Autodesk Fusion 360 part; units mm, degrees
(part 2 of 2)
  spline S18 degree 5 poles (2.4575, 16.735) (2.4592, 16.7471) (2.4624, 16.7712) (2.466, 16.8075) (2.4685, 16.8561) (2.4687, 16.9171) (2.4667, 16.9782) (2.4633, 17.0395) (2.4593, 17.1009) (2.4548, 17.1623) (2.4497, 17.2237) (2.4439, 17.2852) (2.4372, 17.3467) (2.4294, 17.4083) (2.4206, 17.4699) (2.4107, 17.5316) (2.4, 17.5933) (2.3886, 17.6549) (2.3766, 17.7166) (2.364, 17.7783) (2.3508, 17.84) (2.337, 17.9017) (2.3225, 17.9634) (2.3073, 18.025) (2.2914, 18.0867) (2.2749, 18.1483) (2.2578, 18.2099) (2.2401, 18.2715) (2.2219, 18.3331) (2.2031, 18.3946) (2.1837, 18.4561) (2.1638, 18.5175) (2.1433, 18.579) (2.1223, 18.6403) (2.1007, 18.7017) (2.0786, 18.763) (2.056, 18.8242) (2.0329, 18.8854) (2.0092, 18.9465) (1.9851, 19.0076) (1.9605, 19.0686) (1.9353, 19.1296) (1.9097, 19.1905) (1.8836, 19.2514) (1.857, 19.3121) (1.8299, 19.3728) (1.8024, 19.4335) (1.7743, 19.494) (1.7459, 19.5545) (1.7169, 19.615) (1.6875, 19.6753) (1.6577, 19.7355) (1.6274, 19.7957) (1.5966, 19.8558) (1.5654, 19.9158) (1.5338, 19.9757) (1.5017, 20.0356) (1.4692, 20.0953) (1.4362, 20.155) (1.4029, 20.2145) (1.3691, 20.274) (1.3348, 20.3333) (1.3002, 20.3926) (1.2651, 20.4518) (1.2296, 20.5108) (1.1937, 20.5698) (1.1574, 20.6286) (1.1207, 20.6874) (1.0836, 20.746) (1.0461, 20.8045) (1.0082, 20.8629) (0.9775, 20.9095) (0.9544, 20.9445) (0.9388, 20.9677) (0.931, 20.9794) knots 0 0 0 0 0 0 0.01428571 0.02857143 0.04285714 0.05714286 0.07142857 0.08571429 0.1 0.11428571 0.12857143 0.14285714 0.15714286 0.17142857 0.18571429 0.2 0.21428571 0.22857143 0.24285714 0.25714286 0.27142857 0.28571429 0.3 0.31428571 0.32857143 0.34285714 0.35714286 0.37142857 0.38571429 0.4 0.41428571 0.42857143 0.44285714 0.45714286 0.47142857 0.48571429 0.5 0.51428571 0.52857143 0.54285714 0.55714286 0.57142857 0.58571429 0.6 0.61428571 0.62857143 0.64285714 0.65714286 0.67142857 0.68571429 0.7 0.71428571 0.72857143 0.74285714 0.75714286 0.77142857 0.78571429 0.8 0.81428571 0.82857143 0.84285714 0.85714286 0.87142857 0.88571429 0.9 0.91428571 0.92857143 0.94285714 0.95714286 0.97142857 0.98571429 1 1 1 1 1 1
  arc A29 (0.931, 20.9794) -> (-0.931, 20.9794) centre (0, 0) ccw
  spline S19 degree 5 poles (-0.931, 20.9794) (-0.9388, 20.9677) (-0.9544, 20.9445) (-0.9775, 20.9095) (-1.0082, 20.8629) (-1.0461, 20.8045) (-1.0836, 20.746) (-1.1207, 20.6874) (-1.1574, 20.6286) (-1.1937, 20.5698) (-1.2296, 20.5108) (-1.2651, 20.4518) (-1.3002, 20.3926) (-1.3348, 20.3333) (-1.3691, 20.274) (-1.4029, 20.2145) (-1.4362, 20.155) (-1.4692, 20.0953) (-1.5017, 20.0356) (-1.5338, 19.9757) (-1.5654, 19.9158) (-1.5966, 19.8558) (-1.6274, 19.7957) (-1.6577, 19.7355) (-1.6875, 19.6753) (-1.7169, 19.615) (-1.7459, 19.5545) (-1.7743, 19.494) (-1.8024, 19.4335) (-1.8299, 19.3728) (-1.857, 19.3121) (-1.8836, 19.2514) (-1.9097, 19.1905) (-1.9353, 19.1296) (-1.9605, 19.0686) (-1.9851, 19.0076) (-2.0092, 18.9465) (-2.0329, 18.8854) (-2.056, 18.8242) (-2.0786, 18.763) (-2.1007, 18.7017) (-2.1223, 18.6403) (-2.1433, 18.579) (-2.1638, 18.5175) (-2.1837, 18.4561) (-2.2031, 18.3946) (-2.2219, 18.3331) (-2.2401, 18.2715) (-2.2578, 18.2099) (-2.2749, 18.1483) (-2.2914, 18.0867) (-2.3073, 18.025) (-2.3225, 17.9634) (-2.337, 17.9017) (-2.3508, 17.84) (-2.364, 17.7783) (-2.3766, 17.7166) (-2.3886, 17.6549) (-2.4, 17.5933) (-2.4107, 17.5316) (-2.4206, 17.4699) (-2.4294, 17.4083) (-2.4372, 17.3467) (-2.4439, 17.2852) (-2.4497, 17.2237) (-2.4548, 17.1623) (-2.4593, 17.1009) (-2.4633, 17.0395) (-2.4667, 16.9782) (-2.4687, 16.9171) (-2.4685, 16.8561) (-2.466, 16.8075) (-2.4624, 16.7712) (-2.4592, 16.7471) (-2.4575, 16.735) knots -1 -1 -1 -1 -1 -1 -0.98571429 -0.97142857 -0.95714286 -0.94285714 -0.92857143 -0.91428571 -0.9 -0.88571429 -0.87142857 -0.85714286 -0.84285714 -0.82857143 -0.81428571 -0.8 -0.78571429 -0.77142857 -0.75714286 -0.74285714 -0.72857143 -0.71428571 -0.7 -0.68571429 -0.67142857 -0.65714286 -0.64285714 -0.62857143 -0.61428571 -0.6 -0.58571429 -0.57142857 -0.55714286 -0.54285714 -0.52857143 -0.51428571 -0.5 -0.48571429 -0.47142857 -0.45714286 -0.44285714 -0.42857143 -0.41428571 -0.4 -0.38571429 -0.37142857 -0.35714286 -0.34285714 -0.32857143 -0.31428571 -0.3 -0.28571429 -0.27142857 -0.25714286 -0.24285714 -0.22857143 -0.21428571 -0.2 -0.18571429 -0.17142857 -0.15714286 -0.14285714 -0.12857143 -0.11428571 -0.1 -0.08571429 -0.07142857 -0.05714286 -0.04285714 -0.02857143 -0.01428571 0 0 0 0 0 0
  line L19 (-2.4575, 16.735) -> (-2.2515, 15.3323)
  arc A30 (-3.0322, 14.2091) -> (-2.2515, 15.3323) centre (-3.2409, 15.1871) ccw
  arc A31 (-5.7163, 14.4039) -> (-4.4786, 13.8215) centre (-4.7868, 14.7728) ccw
  line L20 (-5.7163, 14.4039) -> (-6.2393, 15.7217)
  spline S20 degree 5 poles (-6.2393, 15.7217) (-6.2438, 15.733) (-6.2531, 15.7555) (-6.2682, 15.7887) (-6.2903, 15.8321) (-6.3206, 15.885) (-6.3529, 15.9369) (-6.3864, 15.9883) (-6.4206, 16.0394) (-6.4553, 16.0903) (-6.4904, 16.141) (-6.5261, 16.1914) (-6.5627, 16.2413) (-6.6002, 16.2907) (-6.6387, 16.3397) (-6.678, 16.3882) (-6.7181, 16.4362) (-6.7588, 16.4839) (-6.8001, 16.5314) (-6.8418, 16.5785) (-6.8841, 16.6253) (-6.927, 16.6718) (-6.9703, 16.718) (-7.0143, 16.7638) (-7.0589, 16.8092) (-7.104, 16.8544) (-7.1496, 16.8992) (-7.1957, 16.9436) (-7.2423, 16.9878) (-7.2894, 17.0317) (-7.3369, 17.0753) (-7.3849, 17.1185) (-7.4333, 17.1615) (-7.4822, 17.2042) (-7.5315, 17.2465) (-7.5813, 17.2885) (-7.6315, 17.3303) (-7.6822, 17.3717) (-7.7332, 17.4128) (-7.7847, 17.4536) (-7.8365, 17.4942) (-7.8888, 17.5344) (-7.9414, 17.5743) (-7.9944, 17.614) (-8.0479, 17.6533) (-8.1017, 17.6923) (-8.1559, 17.7311) (-8.2104, 17.7695) (-8.2653, 17.8077) (-8.3206, 17.8455) (-8.3762, 17.8831) (-8.4322, 17.9203) (-8.4885, 17.9573) (-8.5452, 17.9939) (-8.6022, 18.0303) (-8.6596, 18.0664) (-8.7173, 18.1022) (-8.7753, 18.1376) (-8.8337, 18.1728) (-8.8924, 18.2077) (-8.9514, 18.2423) (-9.0107, 18.2766) (-9.0703, 18.3106) (-9.1303, 18.3443) (-9.1905, 18.3777) (-9.2511, 18.4108) (-9.3119, 18.4436) (-9.3731, 18.4761) (-9.4345, 18.5084) (-9.4963, 18.5403) (-9.5583, 18.5719) (-9.6082, 18.597) (-9.6457, 18.6156) (-9.6708, 18.628) (-9.6834, 18.6342) knots 0 0 0 0 0 0 0.01428571 0.02857143 0.04285714 0.05714286 0.07142857 0.08571429 0.1 0.11428571 0.12857143 0.14285714 0.15714286 0.17142857 0.18571429 0.2 0.21428571 0.22857143 0.24285714 0.25714286 0.27142857 0.28571429 0.3 0.31428571 0.32857143 0.34285714 0.35714286 0.37142857 0.38571429 0.4 0.41428571 0.42857143 0.44285714 0.45714286 0.47142857 0.48571429 0.5 0.51428571 0.52857143 0.54285714 0.55714286 0.57142857 0.58571429 0.6 0.61428571 0.62857143 0.64285714 0.65714286 0.67142857 0.68571429 0.7 0.71428571 0.72857143 0.74285714 0.75714286 0.77142857 0.78571429 0.8 0.81428571 0.82857143 0.84285714 0.85714286 0.87142857 0.88571429 0.9 0.91428571 0.92857143 0.94285714 0.95714286 0.97142857 0.98571429 1 1 1 1 1 1
  arc A32 (-9.6834, 18.6342) -> (-11.296, 17.7031) centre (0, 0) ccw
  spline S21 degree 5 poles (-11.296, 17.7031) (-11.2969, 17.6892) (-11.2987, 17.6613) (-11.3013, 17.6194) (-11.3046, 17.5637) (-11.3082, 17.4942) (-11.3114, 17.4247) (-11.3143, 17.3554) (-11.3167, 17.2862) (-11.3187, 17.2171) (-11.3203, 17.1481) (-11.3215, 17.0792) (-11.3223, 17.0104) (-11.3227, 16.9418) (-11.3226, 16.8733) (-11.3222, 16.8049) (-11.3213, 16.7366) (-11.32, 16.6685) (-11.3183, 16.6005) (-11.3161, 16.5326) (-11.3136, 16.4649) (-11.3106, 16.3973) (-11.3072, 16.3299) (-11.3033, 16.2627) (-11.2991, 16.1955) (-11.2944, 16.1286) (-11.2892, 16.0618) (-11.2836, 15.9952) (-11.2776, 15.9287) (-11.2712, 15.8624) (-11.2643, 15.7963) (-11.2569, 15.7304) (-11.2491, 15.6646) (-11.2408, 15.5991) (-11.2321, 15.5337) (-11.223, 15.4685) (-11.2133, 15.4036) (-11.2032, 15.3388) (-11.1927, 15.2742) (-11.1816, 15.2099) (-11.1701, 15.1458) (-11.1581, 15.0819) (-11.1456, 15.0182) (-11.1327, 14.9548) (-11.1192, 14.8916) (-11.1052, 14.8286) (-11.0907, 14.766) (-11.0758, 14.7035) (-11.0603, 14.6413) (-11.0443, 14.5794) (-11.0278, 14.5178) (-11.0107, 14.4565) (-10.993, 14.3955) (-10.9747, 14.3348) (-10.9559, 14.2745) (-10.9365, 14.2145) (-10.9165, 14.1547) (-10.8961, 14.0953) (-10.8751, 14.0362) (-10.8535, 13.9774) (-10.8312, 13.9191) (-10.8081, 13.8613) (-10.7841, 13.8041) (-10.7591, 13.7475) (-10.7334, 13.6913) (-10.707, 13.6356) (-10.6803, 13.5801) (-10.6531, 13.525) (-10.6253, 13.4703) (-10.5965, 13.4163) (-10.5658, 13.3636) (-10.5393, 13.3228) (-10.5181, 13.2931) (-10.5033, 13.2738) (-10.4957, 13.2642) knots -1 -1 -1 -1 -1 -1 -0.98571429 -0.97142857 -0.95714286 -0.94285714 -0.92857143 -0.91428571 -0.9 -0.88571429 -0.87142857 -0.85714286 -0.84285714 -0.82857143 -0.81428571 -0.8 -0.78571429 -0.77142857 -0.75714286 -0.74285714 -0.72857143 -0.71428571 -0.7 -0.68571429 -0.67142857 -0.65714286 -0.64285714 -0.62857143 -0.61428571 -0.6 -0.58571429 -0.57142857 -0.55714286 -0.54285714 -0.52857143 -0.51428571 -0.5 -0.48571429 -0.47142857 -0.45714286 -0.44285714 -0.42857143 -0.41428571 -0.4 -0.38571429 -0.37142857 -0.35714286 -0.34285714 -0.32857143 -0.31428571 -0.3 -0.28571429 -0.27142857 -0.25714286 -0.24285714 -0.22857143 -0.21428571 -0.2 -0.18571429 -0.17142857 -0.15714286 -0.14285714 -0.12857143 -0.11428571 -0.1 -0.08571429 -0.07142857 -0.05714286 -0.04285714 -0.02857143 -0.01428571 0 0 0 0 0 0
  line L21 (-10.4957, 13.2642) -> (-9.616, 12.1524)
  arc A33 (-9.7305, 10.7893) -> (-9.616, 12.1524) centre (-10.4002, 11.5319) ccw
  arc A34 (-12.1524, 9.616) -> (-10.7893, 9.7305) centre (-11.5319, 10.4002) ccw
  line L22 (-12.1524, 9.616) -> (-13.2642, 10.4957)
  spline S22 degree 5 poles (-13.2642, 10.4957) (-13.2738, 10.5033) (-13.2931, 10.5181) (-13.3228, 10.5393) (-13.3636, 10.5658) (-13.4163, 10.5965) (-13.4703, 10.6253) (-13.525, 10.6531) (-13.5801, 10.6803) (-13.6356, 10.707) (-13.6913, 10.7334) (-13.7475, 10.7591) (-13.8041, 10.7841) (-13.8613, 10.8081) (-13.9191, 10.8312) (-13.9774, 10.8535) (-14.0362, 10.8751) (-14.0953, 10.8961) (-14.1547, 10.9165) (-14.2145, 10.9365) (-14.2745, 10.9559) (-14.3348, 10.9747) (-14.3955, 10.993) (-14.4565, 11.0107) (-14.5178, 11.0278) (-14.5794, 11.0443) (-14.6413, 11.0603) (-14.7035, 11.0758) (-14.766, 11.0907) (-14.8286, 11.1052) (-14.8916, 11.1192) (-14.9548, 11.1327) (-15.0182, 11.1456) (-15.0819, 11.1581) (-15.1458, 11.1701) (-15.2099, 11.1816) (-15.2742, 11.1927) (-15.3388, 11.2032) (-15.4036, 11.2133) (-15.4685, 11.223) (-15.5337, 11.2321) (-15.5991, 11.2408) (-15.6646, 11.2491) (-15.7304, 11.2569) (-15.7963, 11.2643) (-15.8624, 11.2712) (-15.9287, 11.2776) (-15.9952, 11.2836) (-16.0618, 11.2892) (-16.1286, 11.2944) (-16.1955, 11.2991) (-16.2627, 11.3033) (-16.3299, 11.3072) (-16.3973, 11.3106) (-16.4649, 11.3136) (-16.5326, 11.3161) (-16.6005, 11.3183) (-16.6685, 11.32) (-16.7366, 11.3213) (-16.8049, 11.3222) (-16.8733, 11.3226) (-16.9418, 11.3227) (-17.0104, 11.3223) (-17.0792, 11.3215) (-17.1481, 11.3203) (-17.2171, 11.3187) (-17.2862, 11.3167) (-17.3554, 11.3143) (-17.4247, 11.3114) (-17.4942, 11.3082) (-17.5637, 11.3046) (-17.6194, 11.3013) (-17.6613, 11.2987) (-17.6892, 11.2969) (-17.7031, 11.296) knots 0 0 0 0 0 0 0.01428571 0.02857143 0.04285714 0.05714286 0.07142857 0.08571429 0.1 0.11428571 0.12857143 0.14285714 0.15714286 0.17142857 0.18571429 0.2 0.21428571 0.22857143 0.24285714 0.25714286 0.27142857 0.28571429 0.3 0.31428571 0.32857143 0.34285714 0.35714286 0.37142857 0.38571429 0.4 0.41428571 0.42857143 0.44285714 0.45714286 0.47142857 0.48571429 0.5 0.51428571 0.52857143 0.54285714 0.55714286 0.57142857 0.58571429 0.6 0.61428571 0.62857143 0.64285714 0.65714286 0.67142857 0.68571429 0.7 0.71428571 0.72857143 0.74285714 0.75714286 0.77142857 0.78571429 0.8 0.81428571 0.82857143 0.84285714 0.85714286 0.87142857 0.88571429 0.9 0.91428571 0.92857143 0.94285714 0.95714286 0.97142857 0.98571429 1 1 1 1 1 1
  arc A35 (-17.7031, 11.296) -> (-18.6342, 9.6834) centre (0, 0) ccw
  spline S23 degree 5 poles (-18.6342, 9.6834) (-18.628, 9.6708) (-18.6156, 9.6457) (-18.597, 9.6082) (-18.5719, 9.5583) (-18.5403, 9.4963) (-18.5084, 9.4345) (-18.4761, 9.3731) (-18.4436, 9.3119) (-18.4108, 9.2511) (-18.3777, 9.1905) (-18.3443, 9.1303) (-18.3106, 9.0703) (-18.2766, 9.0107) (-18.2423, 8.9514) (-18.2077, 8.8924) (-18.1728, 8.8337) (-18.1376, 8.7753) (-18.1022, 8.7173) (-18.0664, 8.6596) (-18.0303, 8.6022) (-17.9939, 8.5452) (-17.9573, 8.4885) (-17.9203, 8.4322) (-17.8831, 8.3762) (-17.8455, 8.3206) (-17.8077, 8.2653) (-17.7695, 8.2104) (-17.7311, 8.1559) (-17.6923, 8.1017) (-17.6533, 8.0479) (-17.614, 7.9944) (-17.5743, 7.9414) (-17.5344, 7.8888) (-17.4942, 7.8365) (-17.4536, 7.7847) (-17.4128, 7.7332) (-17.3717, 7.6822) (-17.3303, 7.6315) (-17.2885, 7.5813) (-17.2465, 7.5315) (-17.2042, 7.4822) (-17.1615, 7.4333) (-17.1185, 7.3849) (-17.0753, 7.3369) (-17.0317, 7.2894) (-16.9878, 7.2423) (-16.9436, 7.1957) (-16.8992, 7.1496) (-16.8544, 7.104) (-16.8092, 7.0589) (-16.7638, 7.0143) (-16.718, 6.9703) (-16.6718, 6.927) (-16.6253, 6.8841) (-16.5785, 6.8418) (-16.5314, 6.8001) (-16.4839, 6.7588) (-16.4362, 6.7181) (-16.3882, 6.678) (-16.3397, 6.6387) (-16.2907, 6.6002) (-16.2413, 6.5627) (-16.1914, 6.5261) (-16.141, 6.4904) (-16.0903, 6.4553) (-16.0394, 6.4206) (-15.9883, 6.3864) (-15.9369, 6.3529) (-15.885, 6.3206) (-15.8321, 6.2903) (-15.7887, 6.2682) (-15.7555, 6.2531) (-15.733, 6.2438) (-15.7217, 6.2393) knots -1 -1 -1 -1 -1 -1 -0.98571429 -0.97142857 -0.95714286 -0.94285714 -0.92857143 -0.91428571 -0.9 -0.88571429 -0.87142857 -0.85714286 -0.84285714 -0.82857143 -0.81428571 -0.8 -0.78571429 -0.77142857 -0.75714286 -0.74285714 -0.72857143 -0.71428571 -0.7 -0.68571429 -0.67142857 -0.65714286 -0.64285714 -0.62857143 -0.61428571 -0.6 -0.58571429 -0.57142857 -0.55714286 -0.54285714 -0.52857143 -0.51428571 -0.5 -0.48571429 -0.47142857 -0.45714286 -0.44285714 -0.42857143 -0.41428571 -0.4 -0.38571429 -0.37142857 -0.35714286 -0.34285714 -0.32857143 -0.31428571 -0.3 -0.28571429 -0.27142857 -0.25714286 -0.24285714 -0.22857143 -0.21428571 -0.2 -0.18571429 -0.17142857 -0.15714286 -0.14285714 -0.12857143 -0.11428571 -0.1 -0.08571429 -0.07142857 -0.05714286 -0.04285714 -0.02857143 -0.01428571 0 0 0 0 0 0
  line L23 (-15.7217, 6.2393) -> (-14.4039, 5.7163)
  arc A36 (-13.8215, 4.4786) -> (-14.4039, 5.7163) centre (-14.7728, 4.7868) ccw
  circle A37 centre (0, 0) radius 10 construction
  circle A38 centre (-10, 0) radius 2
  arc A39 (-14.2091, -3.0322) -> (-13.8215, -4.4786) centre (0, 0) ccw
  arc A40 (-10.7893, -9.7305) -> (-9.7305, -10.7893) centre (0, 0) ccw
  arc A41 (-4.4786, -13.8215) -> (-3.0322, -14.2091) centre (0, 0) ccw
  arc A42 (3.0322, -14.2091) -> (4.4786, -13.8215) centre (0, 0) ccw
  arc A43 (9.7305, -10.7893) -> (10.7893, -9.7305) centre (0, 0) ccw
  arc A44 (13.8215, -4.4786) -> (14.2091, -3.0322) centre (0, 0) ccw
  arc A45 (14.2091, 3.0322) -> (13.8215, 4.4786) centre (0, 0) ccw
  arc A46 (10.7893, 9.7305) -> (9.7305, 10.7893) centre (0, 0) ccw
  arc A47 (4.4786, 13.8215) -> (3.0322, 14.2091) centre (0, 0) ccw
  arc A48 (-3.0322, 14.2091) -> (-4.4786, 13.8215) centre (0, 0) ccw
  arc A49 (-9.7305, 10.7893) -> (-10.7893, 9.7305) centre (0, 0) ccw
  circle A50 centre (0, 0) radius 1.75
  circle A51 centre (0, 0) radius 3.5
  line L24 (-10, -4) -> (36, -4)
  arc A52 (36, -4) -> (36, 4) centre (36, 0) ccw
  line L25 (36, 4) -> (-10, 4)
  arc A53 (-10, 4) -> (-10, -4) centre (-10, 0) ccw
  line L26 (-10, 0) -> (36, 0) construction
  circle A54 centre (36, 0) radius 2
  dimension "d15" = 20
  dimension "d16" = 4
  dimension "d25" = 7
  dimension "d27" = 8
  dimension "d28" = 4
  dimension "d206" = 46
  constraint coincident A0.centre A2.centre
  constraint coincident A37 A38.centre
  constraint tangent L24 A52
  constraint tangent A52 L25
  constraint parallel L24 L25
  constraint tangent L25 A53
  constraint tangent L24 A53
  constraint horizontal L26
  constraint coincident A38.centre A53.centre
  constraint concentric A52 A54
  measures "d15" diameter of A37
  measures "d16" diameter of A38
  measures "d25" diameter of A51
  measures "d27" diameter of A52
  measures "d28" diameter of A54
  measures "d206" distance of A38.centre A52.centre
extrude "Extrude4" add sketch "Connecting Rod" along normal blind 5 separate body contours A19 L12 S12 A20 S13 L13 A21 A44 A45 L24 A52 L25 | A19 L12 S12 A20 S13 L13 A21 A44 A45 L24 L25 A53 | A50 | A51 makes body 2
extrude "Extrude5" cut sketch "Connecting Rod" against normal blind 3 contours A51 bodies 1
sketch "Slider" plane through (0, 0, 8) normal (0, 0, 1) x (-1, 0, 0)
  line L0 (32, 5) -> (47, 5)
  line L1 (47, 5) -> (47, -5)
  line L2 (47, -5) -> (32, -5)
  line L3 (32, -5) -> (32, 5)
  circle A0 centre (36, 0) radius 2
  point P0 (36, 0)
  dimension "d33" = 10
  dimension "d34" = 15
  dimension "d209" = 4
  constraint horizontal L0
  constraint vertical L1
  constraint horizontal L2
  constraint vertical L3
  measures "d33" distance of L0.end L1.end
  measures "d34" distance of L0.start L0.end
  measures "d209" distance of L3 P0
extrude "Extrude6" add sketch "Slider" against normal blind 8 separate body makes body 3
extrude "Extrude7" add sketch "Connecting Rod" against normal blind 8 contours A54 bodies 3
extrude "Extrude8" add sketch "Connecting Rod" along normal blind 5 contours A38 bodies 1
extrude "Extrude9" add sketch "Connecting Rod" along normal blind 5 contours A54 bodies 3
sketch "Slider Dowel Hole" plane through (-47, 0, 0) normal (-1, 0, 0) x (0, -1, 0)
  line L0 (5, 8) -> (-5, 8)
  line L1 (-5, 8) -> (-5, 0)
  line L2 (-5, 0) -> (5, 0)
  line L3 (5, 0) -> (5, 8)
  line L4 (0, 1.75) -> (0, 22.5)
  circle A0 centre (0, 4) radius 3.1
  point P0 (2.2515, 8)
  dimension "d44" = 6.2
  dimension "d45" = 4
  constraint coincident L4 A0.centre
  measures "d44" diameter of A0
  measures "d45" vertical distance of A0.centre P0
extrude "Extrude10" cut sketch "Slider Dowel Hole" against normal blind 10 contours A0 bodies 3
sketch "Sketch17" plane through (-37, 0, 0) normal (-1, 0, 0) x (0, -1, 0)
  circle A0 centre (0, 4) radius 3.1
  circle A1 centre (0, 4) radius 3.1
  circle A2 centre (0, 4) radius 2.25
  dimension "d213" = 4.5
  constraint concentric A1 A2
  measures "d213" diameter of A2
extrude "Extrude26" cut sketch "Sketch17" against normal blind 5 contours A2 bodies 3
sketch "Connector Rod Clearance" plane through (0, 0, 13) normal (0, 0, 1) x (-1, 0, 0)
  circle A0 centre (-10, 0) radius 2
  circle A1 centre (36, 0) radius 2
  arc A2 (-10, 4) -> (-10, -4) centre (-10, 0) ccw
  line L0 (-10, -4) -> (36, -4)
  arc A3 (36, -4) -> (36, 4) centre (36, 0) ccw
  line L1 (36, 4) -> (-10, 4)
  circle A4 centre (-10, 0) radius 2
  circle A5 centre (36, 0) radius 2
  circle A6 centre (-10, 0) radius 2.15
  circle A7 centre (36, 0) radius 2.15
  dimension "d174" = 4.3
  dimension "d175" = 4.3
  constraint concentric A0 A6
  constraint concentric A1 A7
  measures "d174" diameter of A6
  measures "d175" diameter of A7
ref_plane "WorkPlane1" through (-36, 0, 13.5) normal (0, 0, 1) x (-1, 0, 0)
sketch "Sketch16" plane through (0, 0, 13.5) normal (0, 0, 1) x (1, 0, 0)
  circle A0 centre (-36, 0) radius 2
  circle A1 centre (-36, 0) radius 3
  circle A2 centre (10, 0) radius 2
  circle A3 centre (10, 0) radius 3
  dimension "d187" = 6
  dimension "d188" = 6
  constraint concentric A0 A1
  constraint concentric A2 A3
  measures "d187" diameter of A1
  measures "d188" diameter of A3
extrude "Extrude22" cut sketch "Connector Rod Clearance" against normal blind 5 contours A6 | A7 bodies 2
extrude "Extrude23" add sketch "Sketch16" along normal blind 4 separate body contours A0 | A1 | A2 | A3 makes body 4 at (-33.0149, -0.2987, 14.8333) makes body 5 at (12.9851, -0.2987, 14.8333)
extrude "Extrude24" cut sketch "Connector Rod Clearance" 2 faces at (9.427, 0.4727, 13) (-36.0487, -0.65, 13) along normal blind 2 contours A6 | A7 on bodies 1 3 bodies 4 5
extrude "Extrude33" add 1 faces at (-36.0487, -0.65, 13) along direction (0, 0, 1) blind 2 on bodies 3 bodies 3
extrude "Extrude34" add 1 faces at (9.427, 0.4727, 13) along direction (0, 0, 1) blind 2 on bodies 1 bodies 1
sketch "Base Plate" plane through (0, 0, 0) normal (0, 0, 1) x (1, 0, 0)
  line L0 (30, -25) -> (-71, -25)
  line L1 (-71, -25) -> (-71, 39)
  line L2 (30, 39) -> (30, -25)
  line L3 (-47, -5) -> (-47, 5)
  line L4 (0, 0) -> (17, 0) construction
  circle A0 centre (0, 0) radius 1.5
  line L5 (-22, -5.3) -> (-70, -5.3)
  line L6 (-70, -5.3) -> (-70, -10.3)
  line L7 (-70, -10.3) -> (-22, -10.3)
  line L8 (-22, -10.3) -> (-22, -5.3)
  line L9 (-32, -5) -> (-47, -5)
  line L10 (-32, 5) -> (-32, -5)
  line L11 (-22, 5.3) -> (-70, 5.3)
  line L12 (-70, 5.3) -> (-70, 10.3)
  line L13 (-70, 10.3) -> (-22, 10.3)
  line L14 (-22, 10.3) -> (-22, 5.3)
  line L15 (-71, 7) -> (-102, 7) construction
  line L16 (-20.5, 39) -> (-20.5, -25) construction
  line L17 (10, 0) -> (-36, 0) construction
  line L18 (0, 0) -> (9.2345, 25.3717) construction
  line L19 (0, 0) -> (27, 0) construction
  circle A1 centre (9.2345, 25.3717) radius 1.5
  line L20 (-71, 39) -> (30, 39)
  line L21 (-23.5, -3.8) -> (-30.5, -3.8)
  line L22 (-30.5, -3.8) -> (-30.5, 3.8)
  line L23 (-30.5, 3.8) -> (-23.5, 3.8)
  line L24 (-23.5, 3.8) -> (-23.5, -3.8)
  line L25 (-71, 39) -> (-71, 7) construction
  line L26 (-71, 29) -> (-72.5, 29)
  line L27 (-72.5, 29) -> (-72.5, 17)
  line L28 (-72.5, 17) -> (-71, 17)
  line L29 (-71, 17) -> (-71, 29)
  line L30 (30, -15) -> (31.5, -15)
  line L31 (31.5, -15) -> (31.5, -3)
  line L32 (31.5, -3) -> (30, -3)
  line L33 (30, -3) -> (30, -15)
  circle A2 centre (9.2345, 25.3717) radius 12 construction
  arc A3 (20.9794, -0.931) -> (20.9794, 0.931) centre (0, 0) ccw
  dimension "d48" = 25
  dimension "d53" = 3
  dimension "d55" = 0.3
  dimension "d57" = 10
  dimension "d59" = 5
  dimension "d198" = 27
  dimension "d199" = 70
  dimension "d200" = 3
  dimension "d210" = 23
  dimension "d211" = 1
  dimension "d216" = 1.5
  dimension "d217" = 1.5
  dimension "d218" = 1.5
  dimension "d219" = 1.5
  dimension "d220" = 7
  dimension "d221" = 7.6
  dimension "d226" = 64
  dimension "d227" = 13.6283
  dimension "d236" = 32
  dimension "d237" = 1.5
  dimension "d238" = 12
  dimension "d246" = 10
  dimension "d247" = 1.5
  dimension "d248" = 12
  dimension "d249" = 10
  dimension "d283" = 24
  dimension "d318" = 30
  dimension "motor_gear_to_bottom" = 20.7655
  constraint horizontal L0
  constraint vertical L1
  constraint vertical L2
  constraint coincident L4.start A0.centre
  constraint horizontal L4
  constraint horizontal L5
  constraint vertical L6
  constraint horizontal L7
  constraint vertical L8
  constraint symmetric L4 L5.start L11.start
  constraint symmetric L4 L5.end L11.end
  constraint symmetric L4 L6.end L12.end
  constraint symmetric L4 L7.end L13.end
  constraint midpoint L1 L15.start
  constraint perpendicular L1 L15
  constraint midpoint L0 L16.end
  constraint horizontal L19
  constraint coincident L18.end A1.centre
  constraint horizontal L21
  constraint vertical L22
  constraint horizontal L23
  constraint vertical L24
  constraint horizontal L20
  constraint coincident L1.end L20.start
  constraint coincident L2.start L20.end
  constraint coincident L0.start L2.end
  constraint perpendicular L11 L25
  constraint horizontal L26
  constraint vertical L27
  constraint horizontal L28
  constraint vertical L29
  constraint coincident L25 L26.start
  constraint horizontal L30
  constraint vertical L31
  constraint horizontal L32
  constraint vertical L33
  constraint coincident L2 L30.start
  constraint concentric A1 A2
  measures "d48" distance of L0 L4.start
  measures "d53" diameter of A0
  measures "d55" distance of L5 L9
  measures "d57" distance of L8 L10
  measures "d59" distance of L5.end L6.end
  measures "d198" distance of L4.start L18.end
  measures "d199" angle of L18 L19
  measures "d200" diameter of A1
  measures "d210" distance of L3 L6
  measures "d211" distance of L1 L11.end
  measures "d216" distance of L5 L21
  measures "d217" distance of L11 L23
  measures "d218" distance of L8 L24
  measures "d219" distance of L10 L22
  measures "d220" distance of L22.end L23.end
  measures "d221" distance of L21.end L22.end
  measures "d226" distance of L0.start L2.start
  measures "d227" distance of L18.end L20
  measures "d236" distance of L1.end L15.start
  measures "d237" distance of L26.start L26.end
  measures "d238" distance of L26.start L28.end
  measures "d246" distance of L20 L26
  measures "d247" distance of L30.start L30.end
  measures "d248" distance of L30.start L32.end
  measures "d249" distance of L0 L30
  measures "d283" diameter of A2
  measures "d318" distance of L2 L4.start
  measures "motor_gear_to_bottom" distance of L2 L18.end
extrude "Extrude11" add sketch "Base Plate" along normal blind 7.7 separate body contours L5 L6 L7 L8 | L11 L12 L13 L14 makes body 6 at (-38, -10.3, 5.1333) makes body 7 at (-54, 5.3, 5.1333)
extrude "Extrude12" add sketch "Base Plate" against normal blind 3 separate body contours L0 L1 L2 L20 L29 L33 | L2 L30 L31 L32 L33 | L1 L26 L27 L28 L29 | L5 L6 L7 L8 | L11 L12 L13 L14 makes body 8
combine "Combine1" operation add target body 6 tool bodies 7 8
sketch "Top Plate" plane through (-71, 0, 0) normal (-1, 0, 0) x (0, -1, 0)
  line L0 (0, 4) -> (0, 37) construction
  circle A0 centre (0, 37) radius 2.75
  line L1 (0, 4) -> (29, 4) construction
  circle A1 centre (0, -29) radius 2.75
  circle A2 centre (0, 37) radius 4.75
  circle A3 centre (0, -29) radius 4.75
  line L2 (-39, -37.75) -> (-39, 46)
  line L3 (25, 46) -> (25, -37.75)
  line L4 (-17.7031, 7) -> (-13.2642, 7)
  line L5 (-39, -37.75) -> (25, -37.75)
  line L6 (25, 46) -> (-39, 46)
  line L7 (-7, -37.75) -> (-6.796, -5) construction
  line L8 (-30, 0) -> (-37, 0)
  line L9 (25, 0) -> (-18, 0)
  line L10 (25, 0) -> (-17, 0)
  line L11 (-17, 0) -> (-17, -3)
  line L12 (-17, -3) -> (25, -3)
  line L13 (25, -3) -> (25, 0)
  circle A4 centre (0, 4) radius 3.1
  circle A5 centre (0, 4) radius 3.15
  point P0 (0, 4)
  dimension "d77" = 5.5
  dimension "d94" = 9.5
  dimension "d95" = 9.5
  dimension "d130" = 64
  dimension "d309" = 8.75
  dimension "d311" = 46
  dimension "d327" = 33
  dimension "d328" = 33
  dimension "d329" = 6.3
  constraint vertical L0
  constraint coincident L0.end A0.centre
  constraint symmetric A0 L1 A1
  constraint concentric A1 A3
  constraint vertical L2
  constraint vertical L3
  constraint perpendicular L2 L6
  constraint midpoint L5 L7.start
  constraint coincident L3 L9.start
  constraint horizontal L5
  constraint concentric A4 A5
  measures "d77" diameter of A0
  measures "d94" diameter of A2
  measures "d95" diameter of A3
  measures "d130" distance of L3.end L2.start
  measures "d309" distance of A1.centre L5
  measures "d311" distance of L6 L9
  measures "d327" distance of L0.end P0
  measures "d328" distance of A1.centre P0
  measures "d329" diameter of A5
extrude "Extrude13" add sketch "Top Plate" along normal blind 4 separate body contours A0 | A1 | L2 L3 L5 L6 L9 L10 L11 L12 | L3 L9 L10 L11 L12 L13 makes body 9 at (-72.3333, -2.7363, 36.7262) makes body 10 at (-71, 27.05, 4.0833) makes body 11 at (-72.3333, -2.7363, -29.2738)
extrude "Extrude14" add sketch "Top Plate" along normal blind 8 contours A2 | A3 bodies 9 10 11
sketch "Bottom Plate" plane through (30, 0, 0) normal (1, 0, 0) x (0, 1, 0)
  line L0 (39, -37.75) -> (-25, -37.75)
  line L1 (-25, 46) -> (-25, -37.75)
  line L2 (-25, 46) -> (39, 46)
  line L3 (39, -37.75) -> (39, 46)
extrude "Extrude18" add sketch "Bottom Plate" along normal blind 4 separate body makes body 12
combine "Combine2" operation cut target body 9 tool bodies 6 keep tools
combine "Combine3" operation cut target body 12 tool bodies 6 keep tools
move_face "OffsetFaces1" offset -0.2 1 faces at (31.5, -11, -1) on bodies 12
move_face "OffsetFaces2" offset -0.2 4 faces at (30.5667, -7, 0) (30.5667, -7, -3) (30.5667, -15, -1) (30.5667, -3, -2) on bodies 12
move_face "OffsetFaces3" offset -0.2 1 faces at (-72.5, 25, -1) on bodies 9
move_face "OffsetFaces4" offset -0.2 4 faces at (-71.5667, 29, -1) (-72.1333, 21, -3) (-72.1333, 21, 0) (-72.1333, 17, -1) on bodies 9
sketch "Motor Lifter" plane through (30, 0, 0) normal (-1, 0, 0) x (0, -1, 0)
  line L0 (25, -37.75) -> (25, 46)
  line L1 (25, 46) -> (-39, 46)
  line L2 (-39, -37.75) -> (25, -37.75)
  line L3 (-25.3717, 0) -> (-25.3717, 31) construction
  line L4 (-31.5217, 18.5) -> (-19.2217, 18.5)
  line L5 (-19.2217, 18.5) -> (-19.2217, 43.5)
  line L6 (-19.2217, 43.5) -> (-31.5217, 43.5)
  line L7 (-31.5217, 43.5) -> (-31.5217, 18.5)
  line L8 (-31.5217, 18.5) -> (-19.2217, 43.5) construction
  line L9 (-19.2217, 18.5) -> (-31.5217, 43.5) construction
  line L10 (-19.2217, 18.5) -> (-17.2217, 18.5)
  line L11 (-17.2217, 18.5) -> (-17.2217, 43.5)
  line L12 (-17.2217, 43.5) -> (-19.2217, 43.5)
  line L13 (-19.2217, 43.5) -> (-19.2217, 18.5)
  line L14 (-31.5217, 18.5) -> (-33.5217, 18.5)
  line L15 (-33.5217, 18.5) -> (-33.5217, 43.5)
  line L16 (-33.5217, 43.5) -> (-31.5217, 43.5)
  line L17 (-31.5217, 43.5) -> (-31.5217, 18.5)
  line L18 (-39, 46) -> (-39, -37.75)
  line L19 (4, 16) -> (-3, 16)
  line L20 (-3, 16) -> (-3, 23)
  line L21 (-3, 23) -> (4, 23)
  line L22 (4, 23) -> (4, 16)
  line L23 (-34, -17.75) -> (-19, -17.75)
  line L24 (-19, -17.75) -> (-19, -25.75)
  line L25 (-19, -25.75) -> (-34, -25.75)
  line L26 (-34, -25.75) -> (-34, -17.75)
  point P0 (-25.3717, 0)
  point P1 (-25.3717, 31)
  dimension "d251" = 31
  dimension "d252" = 12.3
  dimension "d253" = 25
  dimension "d254" = 2
  dimension "d255" = 2
  dimension "d312" = 7
  dimension "d313" = 7
  dimension "d314" = 23
  dimension "d333" = 21
  dimension "d380" = 15
  dimension "d381" = 8
  dimension "d382" = 12
  dimension "d383" = 5
  constraint vertical L3
  constraint coincident P0 L3.start
  constraint horizontal L4
  constraint perpendicular L4 L5
  constraint parallel L4 L6
  constraint parallel L5 L7
  constraint coincident L8 P1
  constraint coincident L9 P1
  constraint coincident P1 L3.end
  constraint horizontal L10
  constraint vertical L11
  constraint horizontal L12
  constraint vertical L13
  constraint horizontal L14
  constraint vertical L15
  constraint horizontal L16
  constraint vertical L17
  constraint horizontal L19
  constraint vertical L20
  constraint horizontal L21
  constraint vertical L22
  constraint collinear L6 L16
  constraint collinear L6 L12
  constraint horizontal L23
  constraint vertical L24
  constraint horizontal L25
  constraint vertical L26
  measures "d251" distance of P0 P1
  measures "d252" distance of L5.end L6.end
  measures "d253" distance of L4.start L6.end
  measures "d254" distance of L4.end L10.end
  measures "d255" distance of L4.start L14.end
  measures "d312" distance of L19.start L19.end
  measures "d313" distance of L19.start L21.end
  measures "d314" distance of L1 L21
  measures "d333" distance of L0 L22
  measures "d380" distance of L23.start L23.end
  measures "d381" distance of L23.start L25.end
  measures "d382" distance of L2 L25
  measures "d383" distance of L18 L26
extrude "Extrude19" add sketch "Motor Lifter" along normal blind 15.765 contours L4 L5 L6 L7 L13 L17 bodies 12
extrude "Extrude20" add sketch "Motor Lifter" along normal blind 26.765 contours L7 L14 L15 L16 L17 | L5 L10 L11 L12 L13 bodies 12
extrude "Extrude37" cut sketch "Motor Lifter" against normal blind 4 contours L19 L20 L21 L22 | L23 L24 L25 L26 bodies 12
sketch "Top Plate Attachment" plane through (-71, 0, 0) normal (-1, 0, 0) x (0, -1, 0)
  circle A0 centre (0, -16.5) radius 4.75
  circle A1 centre (0, 3.5) radius 3
  line L0 (25, -3) -> (22, -3) construction
  circle A2 centre (0, 3.5) radius 3
  line L1 (-33, 0) -> (-35, 0) construction
  line L2 (25, 0) -> (-17, 0)
  line L3 (-17, 0) -> (-17, -3)
  line L4 (-17, -3) -> (25, -3)
  line L5 (25, -3) -> (25, 0)
  line L6 (-29.2, -3.2) -> (-16.8, -3.2)
  line L7 (-16.8, -3.2) -> (-16.8, 0.2)
  line L8 (-16.8, 0.2) -> (-29.2, 0.2)
  line L9 (-29.2, 0.2) -> (-29.2, -3.2)
  line L10 (25, 46) -> (25, -37.75)
  line L11 (25, -37.75) -> (-39, -37.75)
  circle A3 centre (0, -29) radius 4.75
  circle A4 centre (0, 37) radius 4.75
  line L12 (-39, -37.75) -> (25, -37.75)
  line L13 (25, -37.75) -> (25, 46)
  line L14 (25, 46) -> (-39, 46)
  line L15 (-39, 46) -> (-39, -37.75)
  line L16 (-7, 46) -> (-7, -37.75) construction
  circle A5 centre (20, 1.5) radius 1.4
  circle A6 centre (0, 4) radius 3.15
  circle A7 centre (0, 4) radius 3.15
  circle A8 centre (20, 1.5) radius 3
  line L17 (25, 0) -> (-39, 0)
  line L18 (25, -37.75) -> (25, 46)
  circle A9 centre (-34, 1.5) radius 1.4
  circle A10 centre (-34, 1.5) radius 3
  dimension "d259" = 3
  dimension "d301" = 2.8
  dimension "d330" = 6
  dimension "d331" = 1.5
  dimension "d332" = 5
  constraint horizontal L0
  constraint midpoint L14 L16.start
  constraint midpoint L12 L16.end
  constraint concentric A5 A8
  constraint symmetric L16 A5 A9
  constraint symmetric L16 A8 A10
  measures "d259" distance of L0.start L0.end
  measures "d301" diameter of A5
  measures "d330" diameter of A8
  measures "d331" distance of A5.centre L17
  measures "d332" distance of A5.centre L18
extrude "Extrude27" add sketch "Top Plate Attachment" against normal blind 8 contours L2 A8 L17 | L17 A10 picked at (17.7837, 0.4294) picked at (-36.2163, 0.4294) bodies 6
sketch "Bottom Tabs" plane through (30, 0, 0) normal (-1, 0, 0) x (0, -1, 0)
  line L0 (-17.2217, 18.5) -> (-33.5217, 18.5)
  line L1 (-33.5217, 18.5) -> (-33.5217, 43.5)
  line L2 (-17.2217, 43.5) -> (-17.2217, 18.5)
  line L3 (25, -37.75) -> (25, 46)
  line L4 (25, 46) -> (-39, 46)
  line L5 (-39, -37.75) -> (25, -37.75)
  line L6 (15.2, -3.2) -> (2.8, -3.2)
  line L7 (2.8, -3.2) -> (2.8, 0.2)
  line L8 (2.8, 0.2) -> (15.2, 0.2)
  line L9 (15.2, 0.2) -> (15.2, -3.2)
  line L10 (25, 0) -> (-39, 0)
  line L11 (-31.4019, 0) -> (-36.5981, 0)
  line L12 (-39, 46) -> (-39, -37.75)
  line L13 (-33.5217, 43.5) -> (-17.2217, 43.5)
  line L14 (-3, 16) -> (-3, 23)
  line L15 (-3, 23) -> (4, 23)
  line L16 (4, 23) -> (4, 16)
  line L17 (4, 16) -> (-3, 16)
  line L18 (-31.4019, 0) -> (-36.5981, 0)
  arc A0 (-31.4019, 0) -> (-36.5981, 0) centre (-34, 1.5) ccw
  arc A1 (22.5981, 0) -> (17.4019, 0) centre (20, 1.5) ccw
  circle A2 centre (-34, 1.5) radius 1.4
  arc A3 (-31.4019, 0) -> (-36.5981, 0) centre (-34, 1.5) ccw
  circle A4 centre (20, 1.5) radius 1.4
  line L19 (22.5981, 0) -> (17.4019, 0)
  circle A5 centre (-34, 1.5) radius 1.4
  circle A6 centre (20, 1.5) radius 1.4
  arc A7 (22.5981, 0) -> (17.4019, 0) centre (20, 1.5) ccw
  line L20 (22.5981, 0) -> (17.4019, 0)
  line L21 (-19, -17.75) -> (-19, -25.75)
  line L22 (-19, -25.75) -> (-34, -25.75)
  line L23 (-34, -25.75) -> (-34, -17.75)
  line L24 (-34, -17.75) -> (-19, -17.75)
extrude "Extrude28" add sketch "Bottom Tabs" along normal blind 8 contours L10 A1 L19 A7 L20 | L10 L11 L18 A0 A3 bodies 6
sketch "Sketch20" plane through (34, 0, 0) normal (1, 0, 0) x (0, 1, 0)
  line L0 (-25, 46) -> (-25, -37.75)
  line L1 (-25, -37.75) -> (39, -37.75)
  line L2 (39, -37.75) -> (39, 46)
  line L3 (39, 46) -> (-25, 46)
  circle A0 centre (-20, 1.5) radius 2.5
  circle A1 centre (34, 1.5) radius 2.5
  line L4 (3, 23) -> (3, 16)
  line L5 (3, 16) -> (-4, 16)
  line L6 (-4, 16) -> (-4, 23)
  line L7 (-4, 23) -> (3, 23)
  circle A2 centre (34, 1.5) radius 1.4
  circle A3 centre (-20, 1.5) radius 1.4
  line L8 (19, -25.75) -> (19, -17.75)
  line L9 (19, -17.75) -> (34, -17.75)
  line L10 (34, -17.75) -> (34, -25.75)
  line L11 (34, -25.75) -> (19, -25.75)
  point P0 (-25, 0)
  dimension "d271" = 5
  dimension "d272" = 5
  constraint concentric A0 A3
  constraint concentric A1 A2
  measures "d271" diameter of A0
  measures "d272" diameter of A1
extrude "Extrude29" cut sketch "Sketch20" against normal blind 3 contours A0 | A1 bodies 12
extrude "Extrude30" cut 2 faces at (34, 33.9651, 1.8429) (34, -20.2845, 1.9516) along direction (-1, 0, 0) blind 4 on bodies 12 bodies 12
sketch "Sketch21" plane through (-75, 0, 0) normal (-1, 0, 0) x (0, -1, 0)
  circle A0 centre (-34, 1.5) radius 2.5
  circle A1 centre (20, 1.5) radius 2.5
  circle A2 centre (20, 1.5) radius 1.4
  circle A3 centre (-34, 1.5) radius 1.4
  dimension "d277" = 5
  dimension "d278" = 5
  constraint concentric A0 A3
  constraint concentric A1 A2
  measures "d277" diameter of A0
  measures "d278" diameter of A1
extrude "Extrude31" cut sketch "Sketch21" against normal blind 3 bodies 9
extrude "Extrude32" cut 2 faces at (-75, 34.0349, 1.8429) (-75, -20.5406, 1.1214) along direction (1, 0, 0) blind 4 on bodies 9 bodies 9
ref_plane "WorkPlane2" through (44, 7, 4.125) normal (1, 0, 0) x (0, 1, 0)
sketch "Pcb box" plane through (44, 0, 0) normal (1, 0, 0) x (0, 1, 0)
  line L0 (39, -37.75) -> (39, 46)
  line L1 (-25, -37.75) -> (39, -37.75)
  line L2 (-25, 46) -> (-25, -37.75)
  line L3 (39, 46) -> (-25, 46)
  line L4 (39, 20) -> (54.5, 20)
  line L5 (54.5, 20) -> (54.5, -12)
  line L6 (54.5, -12) -> (39, -12)
  line L7 (39, -12) -> (39, 20)
  line L8 (-9, 46) -> (23, 46)
  line L9 (23, 46) -> (23, 61.5)
  line L10 (23, 61.5) -> (-9, 61.5)
  line L11 (-9, 61.5) -> (-9, 46)
  line L12 (-25, 20) -> (-40.5, 20)
  line L13 (-40.5, 20) -> (-40.5, -12)
  line L14 (-40.5, -12) -> (-25, -12)
  line L15 (-25, -12) -> (-25, 20)
  line L16 (-9, -37.75) -> (23, -37.75)
  line L17 (23, -37.75) -> (23, -53.25)
  line L18 (23, -53.25) -> (-9, -53.25)
  line L19 (-9, -53.25) -> (-9, -37.75)
  line L20 (39, -37.75) -> (31.2, -37.75)
  line L21 (31.2, -37.75) -> (31.2, -29.95)
  line L22 (31.2, -29.95) -> (39, -29.95)
  line L23 (39, -29.95) -> (39, -37.75)
  line L24 (-25, -37.75) -> (-17.2, -37.75)
  line L25 (-17.2, -37.75) -> (-17.2, -29.95)
  line L26 (-17.2, -29.95) -> (-25, -29.95)
  line L27 (-25, -29.95) -> (-25, -37.75)
  line L28 (-25, 46) -> (-17.2, 46)
  line L29 (-17.2, 46) -> (-17.2, 38.2)
  line L30 (-17.2, 38.2) -> (-25, 38.2)
  line L31 (-25, 38.2) -> (-25, 46)
  line L32 (39, 46) -> (31.2, 46)
  line L33 (31.2, 46) -> (31.2, 38.2)
  line L34 (31.2, 38.2) -> (39, 38.2)
  line L35 (39, 38.2) -> (39, 46)
  line L36 (-25, 38.2) -> (-17.2, 46) construction
  line L37 (-25, 46) -> (-17.2, 38.2) construction
  line L38 (31.2, 38.2) -> (39, 46) construction
  line L39 (31.2, 46) -> (39, 38.2) construction
  line L40 (31.2, -29.95) -> (39, -37.75) construction
  line L41 (31.2, -37.75) -> (39, -29.95) construction
  line L42 (-17.2, -29.95) -> (-25, -37.75) construction
  line L43 (-25, -29.95) -> (-17.2, -37.75) construction
  circle A0 centre (-21.1, 42.1) radius 1.4
  circle A1 centre (35.1, 42.1) radius 1.4
  circle A2 centre (-21.1, -33.85) radius 1.4
  circle A3 centre (35.1, -33.85) radius 1.4
  circle A4 centre (-21.1, 42.1) radius 2.5
  circle A5 centre (35.1, 42.1) radius 2.5
  circle A6 centre (35.1, -33.85) radius 2.5
  circle A7 centre (-21.1, -33.85) radius 2.5
  dimension "d335" = 15.5
  dimension "d336" = 32
  dimension "d337" = 26
  dimension "d338" = 32
  dimension "d339" = 15.5
  dimension "d340" = 16
  dimension "d341" = 15.5
  dimension "d342" = 32
  dimension "d343" = 26
  dimension "d344" = 32
  dimension "d345" = 15.5
  dimension "d346" = 16
  dimension "d347" = 7.8
  dimension "d348" = 7.8
  dimension "d349" = 7.8
  dimension "d350" = 7.8
  dimension "d351" = 7.8
  dimension "d352" = 7.8
  dimension "d353" = 7.8
  dimension "d354" = 7.8
  dimension "d355" = 2.8
  dimension "d356" = 2.8
  dimension "d357" = 2.8
  dimension "d358" = 2.8
  dimension "d359" = 5
  dimension "d360" = 5
  dimension "d361" = 5
  dimension "d362" = 5
  constraint horizontal L4
  constraint vertical L5
  constraint horizontal L6
  constraint vertical L7
  constraint coincident L0 L4.start
  constraint horizontal L8
  constraint vertical L9
  constraint horizontal L10
  constraint vertical L11
  constraint coincident L3 L8.start
  constraint horizontal L12
  constraint vertical L13
  constraint horizontal L14
  constraint vertical L15
  constraint coincident L2 L12.start
  constraint horizontal L16
  constraint vertical L17
  constraint horizontal L18
  constraint vertical L19
  constraint coincident L1 L16.start
  constraint horizontal L20
  constraint vertical L21
  constraint horizontal L22
  constraint vertical L23
  constraint coincident L0.start L1.end
  constraint horizontal L24
  constraint vertical L25
  constraint horizontal L26
  constraint vertical L27
  constraint coincident L1.start L2.end
  constraint horizontal L28
  constraint vertical L29
  constraint horizontal L30
  constraint vertical L31
  constraint coincident L2.start L3.end
  constraint horizontal L32
  constraint vertical L33
  constraint horizontal L34
  constraint vertical L35
  constraint coincident L0.end L3.start
  constraint midpoint L37 A0.centre
  constraint midpoint L38 A1.centre
  constraint midpoint L42 A2.centre
  constraint midpoint L41 A3.centre
  constraint concentric A0 A4
  constraint concentric A1 A5
  constraint concentric A3 A6
  constraint concentric A2 A7
  measures "d335" distance of L4.start L4.end
  measures "d336" distance of L4.start L6.end
  measures "d337" distance of L3 L4
  measures "d338" distance of L8.start L8.end
  measures "d339" distance of L8.start L10.end
  measures "d340" distance of L2 L11
  measures "d341" distance of L12.start L12.end
  measures "d342" distance of L12.start L14.end
  measures "d343" distance of L3 L12
  measures "d344" distance of L16.start L16.end
  measures "d345" distance of L16.start L18.end
  measures "d346" distance of L2 L19
  measures "d347" distance of L0.start L20.end
  measures "d348" distance of L0.start L22.end
  measures "d349" distance of L1.start L24.end
  measures "d350" distance of L1.start L26.end
  measures "d351" distance of L2.start L28.end
  measures "d352" distance of L2.start L30.end
  measures "d353" distance of L0.end L32.end
  measures "d354" distance of L0.end L34.end
  measures "d355" diameter of A0
  measures "d356" diameter of A1
  measures "d357" diameter of A2
  measures "d358" diameter of A3
  measures "d359" diameter of A4
  measures "d360" diameter of A5
  measures "d361" diameter of A6
  measures "d362" diameter of A7
extrude "Extrude38" add sketch "Pcb box" along normal blind 2 separate body contours L0 L1 L2 L3 L7 L8 L15 L16 L21 L22 L25 L26 L29 L30 L33 L34 | L0 L4 L5 L6 L7 | L1 L16 L17 L18 L19 | L3 L8 L9 L10 L11 | L2 L12 L13 L14 L15 makes body 13
extrude "Extrude40" add sketch "Pcb box" along normal blind -10 and the other way blind -2 contours L0 L1 L20 L21 L22 L23 | L0 L3 L32 L33 L34 L35 | L1 L2 L24 L25 L26 L27 | L2 L3 L28 L29 L30 L31 | A4 | A5 | A6 | A7 bodies 13
sketch "pcb box holes" plane through (30, 0, 0) normal (-1, 0, 0) x (0, -1, 0)
  circle A0 centre (-34, 1.5) radius 1.4
  circle A1 centre (20, 1.5) radius 1.4
  line L0 (-3, 16) -> (-3, 23)
  line L1 (-3, 23) -> (4, 23)
  line L2 (4, 23) -> (4, 16)
  line L3 (4, 16) -> (-3, 16)
  line L4 (-17.2217, 18.5) -> (-33.5217, 18.5)
  line L5 (-33.5217, 18.5) -> (-33.5217, 43.5)
  line L6 (-33.5217, 43.5) -> (-17.2217, 43.5)
  line L7 (-17.2217, 43.5) -> (-17.2217, 18.5)
  line L8 (25, -37.75) -> (25, 46)
  line L9 (25, 46) -> (-39, 46)
  line L10 (-39, 46) -> (-39, -37.75)
  line L11 (-39, -37.75) -> (25, -37.75)
  line L12 (15.2, -3.2) -> (2.8, -3.2)
  line L13 (2.8, -3.2) -> (2.8, 0.2)
  line L14 (2.8, 0.2) -> (15.2, 0.2)
  line L15 (15.2, 0.2) -> (15.2, -3.2)
  circle A2 centre (-35.1, 42.1) radius 1.4
  circle A3 centre (-35.1, 42.1) radius 2.5
  circle A4 centre (21.1, 42.1) radius 1.4
  circle A5 centre (21.1, 42.1) radius 2.5
  circle A6 centre (21.1, -33.85) radius 2.5
  circle A7 centre (21.1, -33.85) radius 1.4
  circle A8 centre (-35.1, -33.85) radius 2.5
  circle A9 centre (-35.1, -33.85) radius 1.4
  line L16 (-19, -17.75) -> (-19, -25.75)
  line L17 (-19, -25.75) -> (-34, -25.75)
  line L18 (-34, -25.75) -> (-34, -17.75)
  line L19 (-34, -17.75) -> (-19, -17.75)
extrude "Extrude43" cut sketch "pcb box holes" against normal blind 17 contours A4 | A7 | A9 bodies 12
extrude "Extrude44" cut sketch "pcb box holes" against normal blind 3 contours A5 | A6 | A8 bodies 12 13
hidden bodies 1 2 3 4 5 6 9
equation "d1 = thickness"
equation "d3 = thickness"
equation "d16 = peg_diameter"
equation "screw_hole_diam = 3.5 mm"
equation "screw_inset = 3 mm"
equation "wing_movement = 20 mm"
equation "root_fillet = 1 mm"
equation "module = 3"
equation "d22 = screw_hole_diam"
equation "thickness = 8 mm"
equation "inset_diameter = 7 mm"
equation "d25 = inset_diameter"
equation "peg_diameter = 4 mm"
equation "d28 = peg_diameter"
equation "d29 = connector_thickness"
equation "d31 = -screw_inset"
equation "d35 = -thickness"
equation "d37 = -thickness"
equation "connector_thickness = 5 mm"
equation "d40 = connector_thickness"
equation "d42 = connector_thickness"
equation "d44 = tubing_outer_diameter + press_fit_tolerance"
equation "d45 = thickness / 2"
equation "d53 = backing_screw_hole_diam"
equation "d55 = slider_clearence"
equation "slider_clearence = 0.3 mm"
equation "d60 = thickness - slider_clearence"
equation "dowel_hole_diameter = 5.5 mm"
equation "d77 = dowel_hole_diameter"
equation "dowel_hole_wall = 2 mm"
equation "base_width = 64 mm"
equation "base_height = 120 mm"
equation "base_length = 74 mm"
equation "wall_thickness = 3 mm"
equation "d92 = wall_thickness + 1 mm"
equation "d94 = dowel_hole_diameter + 2 * dowel_hole_wall"
equation "d95 = dowel_hole_diameter + 2 * dowel_hole_wall"
equation "dowel_hole_height = 5 mm"
equation "d97 = dowel_hole_height + wall_thickness"
equation "d130 = base_width"
equation "d157 = wall_thickness + 1 mm"
equation "d165 = lifter_height"
equation "d167 = lifter_height + 11 mm"
equation "backing_screw_hole_diam = 3 mm"
equation "d174 = peg_diameter + 0.3 mm"
equation "d175 = peg_diameter + 0.3 mm"
equation "d176 = -connector_thickness"
equation "d187 = cap_size"
equation "d188 = cap_size"
equation "cap_size = 6 mm"
equation "d200 = backing_screw_hole_diam"
equation "d206 = connecting_rod_length"
equation "connecting_rod_length = 46 mm"
equation "d226 = base_width"
equation "tab_height = 1.5 mm"
equation "d236 = base_width / 2"
equation "d237 = tab_height"
equation "tab_clearence = 0.2 mm"
equation "d242 = -tab_clearence"
equation "d243 = -tab_clearence"
equation "d244 = -tab_clearence"
equation "d245 = -tab_clearence"
equation "d247 = tab_height"
equation "d251 = motor_gear_height + motor_length / 2 + 1.5 mm"
equation "lifter_height = 20.765 mm - motor_height / 2"
equation "m3_bolt_width = 2.8 mm"
equation "m3_bolt_cap_diameter = 5 mm"
equation "d271 = m3_bolt_cap_diameter"
equation "d272 = m3_bolt_cap_diameter"
equation "d277 = m3_bolt_cap_diameter"
equation "d278 = m3_bolt_cap_diameter"
equation "nut_tolerance = 0.15 mm"
equation "nut_diameter = 5.35 mm"
equation "nut_thickness = 2.3 mm"
equation "d301 = m3_bolt_width"
equation "wire_to_center_distance = 33 mm"
equation "d309 = 4 mm + dowel_hole_diameter / 2 + dowel_hole_wall"
equation "d316 = -wall_thickness - 1 mm"
equation "motor_height = 10 mm"
equation "motor_width = 12 mm"
equation "press_fit_tolerance = 0.2 mm"
equation "tubing_outer_diameter = 6 mm"
equation "motor_gear_height = 17.5 mm"
equation "motor_length = 24 mm"
equation "d334 = pcb_base_to_base"
equation "d347 = 8 mm - press_fit_tolerance"
equation "d348 = 8 mm - press_fit_tolerance"
equation "d349 = 8 mm - press_fit_tolerance"
equation "d350 = 8 mm - press_fit_tolerance"
equation "d351 = 8 mm - press_fit_tolerance"
equation "d352 = 8 mm - press_fit_tolerance"
equation "d353 = 8 mm - press_fit_tolerance"
equation "d354 = 8 mm - press_fit_tolerance"
equation "d355 = m3_bolt_width"
equation "d356 = m3_bolt_width"
equation "d357 = m3_bolt_width"
equation "d358 = m3_bolt_width"
equation "d359 = m3_bolt_cap_diameter"
equation "d360 = m3_bolt_cap_diameter"
equation "d361 = m3_bolt_cap_diameter"
equation "d362 = m3_bolt_cap_diameter"
equation "d367 = -pcb_base_to_base"
equation "d377 = -screw_inset"
equation "pcb_base_to_base = 10 mm"
named bodies: "Spur Gear (12 teeth)", "Connecting Rod", "Slider", "Base Plate", "Bottom Plate", "Top Plate", "Cap 1", "Cap 2", "PcbBox"
